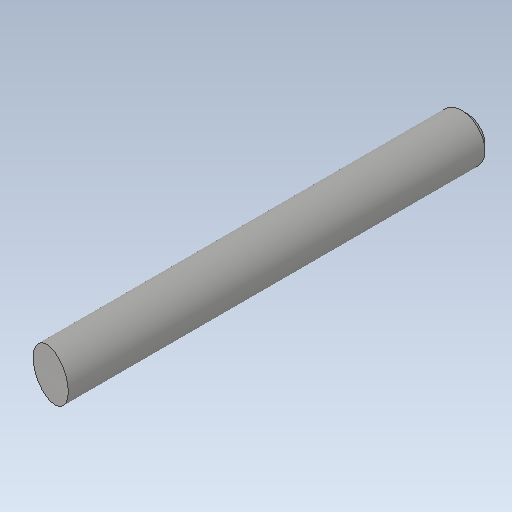
# Autodesk Inventor part: trappestift skrå
Saved by Autodesk Inventor 2020.1 (Build 241239000, 239)
## iProperties
Created: 2019-09-29
Part Number: trappestift skrå
Material: S355J2
Document SubType Name: Modeling
Designer: loppen
Density: 7.85 g/cm^3
Appearance: Light Gray
Mass: 852.536 g
Surface Area: 182.758 cm^2
Volume: 108.603 cm^3
Author: loppen
Autodesk Inventor part; units mm, degrees
ref_plane "YZ Plane" through (0, 0, 0) normal (1, 0, 0) x (0, 1, 0)
ref_plane "XZ Plane" through (0, 0, 0) normal (0, 1, 0) x (-1, 0, 0)
ref_plane "XY Plane" through (0, 0, 0) normal (0, 0, 1) x (1, 0, 0)
sketch "Sketch1" plane through (0, 0, 0) normal (0, 0, 1) x (1, 0, 0)
  circle A0 centre (0, 0) radius 12.5
  dimension "d0" = 25
  constraints: 1 centre point, 1 coincident
  measures "d0" diameter of A0
extrude "Extrusion1" add sketch "Sketch1" along normal blind 228
sketch "Sketch2" plane through (0, 0, 0) normal (0, 1, 0) x (-1, 0, 0)
  line L0 (12.5, 228) -> (-12.5, 228) projected
  line L1 (-12.5, 0) -> (12.5, 0) projected
  line L2 (12.5, 0) -> (12.5, 228) projected
  line L3 (12.5, 228) -> (-12.5, 228) projected
  line L4 (12.5, 221.7204) -> (-12.5, 228)
  point P0 (0, 0)
  dimension "d5" = 14.1
  constraints: 2 end point, 1 point on line
  measures "d5" angle of L4 L0
extrude "Extrusion2" cut sketch "Sketch2" along normal through all both and the other way through all
sketch "Sketch3" plane through (0, 0, 0) normal (0, 1, 0) x (-1, 0, 0)
  line L0 (12.5, 0) -> (12.5, 221.7204) projected
  line L1 (-12.5, 0) -> (-12.5, 228) projected
  line L2 (-12.5, 0) -> (12.5, 0) projected
  line L3 (12.5, 2.953) -> (-12.5, 2.953)
  line L4 (-12.5, 2.953) -> (-12.5, 0)
  line L5 (-12.5, 0) -> (12.5, 0)
  line L6 (12.5, 0) -> (12.5, 2.953)
  point P0 (0, 0)
  dimension "d6" = 2.953
  constraints: 8 end point, 2 parallel, 1 horizontal, 1 perpendicular, 1 point on line
  measures "d6" distance between parallel lines of L2 L3
extrude "Extrusion3" cut sketch "Sketch3" along normal through all both and the other way through all
chamfer "Chamfer1" distance 3 angle 45 1 edges at (-12.5, 0, 2.953)
equation "\"d0\" = trappestifter_dia"
equation "\"d1\" = trappestifter_laengde"
equation "\"trappestifter_dia\" = 25"
equation "\"trappestifter_laengde\" = 228"
equation "\"perforeringsbredde\" = 6"
equation "\"perforeringshullaengde\" = 62.8"
equation "\"perforeringsoffset\" = 8"
equation "\"perforeringsoffset_top\" = 8"
equation "\"perforeringsoffset_bund\" = 8"
equation "\"laskehul_dia\" = 13"
equation "\"perforeringshullaengde_bund\" = 61.6"
equation "\"perforeringshullaengde_top\" = 61"
equation "\"trappestifter_huldia\" = 25.8"
equation "\"trappestifter_skraa_huldia\" = 26.6"
equation "\"trappevinkel\" = 34.3deg"
equation "\"balusterhul_udvidelse\" = 1"
equation "\"pladetykkelse\" = 3"
equation "\"trinbredde\" = 1884"
body "Solid1"
